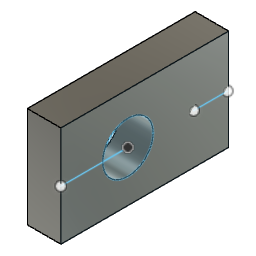
Plate w hole v2 (Autodesk Fusion 360 design; units mm, degrees)
Autodesk Fusion 360 part; units mm, degrees
sketch "Sketch1" plane through (0, 0, 0) normal (1, 0, 0) x (0, 1, 0)
  line L0 (0, 0) -> (31.75, 0)
  line L1 (31.75, 0) -> (31.75, -19.05)
  line L2 (31.75, -19.05) -> (0, -19.05)
  line L3 (0, -19.05) -> (0, 0)
  dimension "d1" = 31.75
  dimension "d2" = 19.05
  constraint horizontal L0
  constraint vertical L1
  constraint horizontal L2
  constraint vertical L3
  constraint coincident L0.start L3.end
  measures "d1" distance of L0.start L0.end
  measures "d2" distance of L0.start L2.end
extrude "Extrude1" add sketch "Sketch1" along normal blind 6.35
sketch "Sketch2" plane through (6.35, 0, 0) normal (1, 0, 0) x (0, 1, 0)
  line L0 (0, -19.05) -> (31.75, -19.05)
  line L1 (31.75, -19.05) -> (31.75, 0)
  line L2 (31.75, 0) -> (0, 0)
  line L3 (0, 0) -> (0, -19.05)
sketch "Sketch3" plane through (6.35, 15.875, -9.525) normal (1, 0, 0) x (0, 1, 0)
  line L0 (15.5884, -0.1633) -> (9.2384, -0.1633)
  line L1 (-15.8946, -0.0015) -> (-3.1946, -0.0015)
  circle A0 centre (-3.1946, -0.0015) radius 4.7625
  dimension "d9" = 6.35
  dimension "d10" = 12.7
  dimension "d11" = 9.525
  constraint horizontal L0
  constraint horizontal L1
  constraint coincident L1.end A0.centre
  measures "d9" distance of L0.start L0.end
  measures "d10" distance of L1.start L1.end
  measures "d11" diameter of A0
hole "Hole3" at (6.35, 12.6804, -9.5265) direction (-1, 0, 0) diameter 9.525 depth 50.8 tip angle 118
